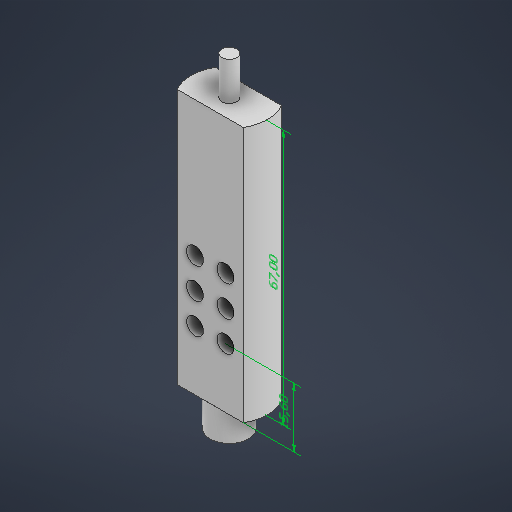
# Autodesk Inventor part: Launcher_shaft
Saved by Autodesk Inventor 2026.1 (Build 301233020, 233B)
## iProperties
Created: 2025-10-31
Part Number: Launcher_shaft
Material: Generic
Document SubType Name: Modeling
Designer: Asus
Density: 1 g/cm^3
Appearance: Default
Author: Asus
Autodesk Inventor part; units mm, degrees
ref_plane "YZ Plane" through (0, 0, 0) normal (1, 0, 0) x (0, 1, 0)
ref_plane "XZ Plane" through (0, 0, 0) normal (0, 1, 0) x (-1, 0, 0)
ref_plane "XY Plane" through (0, 0, 0) normal (0, 0, 1) x (1, 0, 0)
sketch "Sketch1" plane through (0, 0, 0) normal (0, 1, 0) x (-1, 0, 0)
  line L0 (-2.0347, 1.85) -> (2.0347, 1.85)
  line L1 (2.0347, -1.85) -> (-2.0347, -1.85)
  line L2 (-2.0347, 1.85) -> (2.0347, -1.85) construction
  line L3 (2.0347, 1.85) -> (-2.0347, -1.85) construction
  circle A0 centre (0, 0) radius 5
  arc A1 (2.0347, -1.85) -> (2.0347, 1.85) centre (0, 0) ccw
  arc A2 (-2.0347, 1.85) -> (-2.0347, -1.85) centre (0, 0) ccw
  dimension "d2" = 10
  constraints: 8 end point, 4 point on circle, 3 centre point, 2 coincident, 2 midpoint, 1 horizontal, 1 parallel
  measures "d2" diameter of A0
extrude "Extrusion1" add sketch "Sketch1" along normal blind 8
sketch "Sketch2" plane through (0, 8, 0) normal (0, 1, 0) x (1, 0, 0)
  circle A0 centre (0, 0) radius 10
  dimension "d10" = 20
  constraints: 1 centre point, 1 coincident
  measures "d10" diameter of A0
extrude "Extrusion2" add sketch "Sketch2" along normal blind 67
sketch "Sketch3" plane through (0, 75, 0) normal (0, 1, 0) x (1, 0, 0)
  circle A0 centre (0, 0) radius 1.95
  dimension "d7" = 3.9
  constraints: 1 centre point, 1 coincident
  measures "d7" diameter of A0
extrude "Extrusion3" add sketch "Sketch3" along normal blind 10
sketch "Sketch4" plane through (0, 8, 0) normal (0, -1, 0) x (1, 0, 0)
  circle A0 centre (0, 0) radius 5 projected
  line L0 (0, 5) -> (8.6603, 5)
  line L1 (0, 5) -> (-8.6603, 5)
  line L2 (-8.6603, -5) -> (8.6603, -5)
  arc A1 (-8.6603, -5) -> (8.6603, -5) centre (0, 0) ccw
  arc A2 (8.6603, 5) -> (-8.6603, 5) centre (0, 0) ccw
  constraints: 6 end point, 4 point on circle, 2 centre point, 2 horizontal, 1 coincident, 1 parallel, 1 point on line, 1 vertical alignment, 1 other
extrude "Extrusion4" cut sketch "Sketch4" against normal blind 67 contours L2 A1 | L1 A2 L0
sketch "Sketch5" plane through (-8.6603, 8, 5) normal (0, 0, 1) x (1, 0, 0)
  circle A0 centre (4.66, -0.4) radius 2.2
  line L0 (4.66, -0.4) -> (12.66, -0.4) construction
  line L1 (4.66, -0.4) -> (4.66, 67) construction
  line L2 (17.3205, 67) -> (0, 67) projected
  line L3 (4.66, 7.6) -> (4.66, 75) construction
  circle A1 centre (4.66, 7.6) radius 2.2
  line L4 (4.66, 15.6) -> (4.66, 83) construction
  circle A2 centre (4.66, 15.6) radius 2.2
  line L5 (4.66, 23.6) -> (4.66, 91) construction
  circle A3 centre (4.66, 23.6) radius 2.2
  line L6 (4.66, 31.6) -> (4.66, 99) construction
  circle A4 centre (4.66, 31.6) radius 2.2
  line L7 (12.66, -0.4) -> (12.66, 67) construction
  circle A5 centre (12.66, -0.4) radius 2.2
  line L8 (12.66, 7.6) -> (12.66, 75) construction
  circle A6 centre (12.66, 7.6) radius 2.2
  line L9 (12.66, 15.6) -> (12.66, 83) construction
  circle A7 centre (12.66, 15.6) radius 2.2
  line L10 (12.66, 23.6) -> (12.66, 91) construction
  circle A8 centre (12.66, 23.6) radius 2.2
  line L11 (12.66, 31.6) -> (12.66, 99) construction
  circle A9 centre (12.66, 31.6) radius 2.2
  line L12 (8.6603, 0) -> (0, 0) projected
  line L13 (13.6603, -8) -> (3.6603, -8) projected
  point P0 (8.6603, -8)
  dimension "d24" = 8
  dimension "d27" = 8
  dimension "d33" = 7.6
  constraints: 22 end point, 10 centre point, 2 horizontal, 2 vertical, 1 collinear, 1 point on line, 35 other
  measures "d24" distance of L0.start L3.start
  measures "d27" distance of L0.start L7.start
  measures "d33" distance from line of L13 L0.start
extrude "Extrusion5" cut sketch "Sketch5" against normal blind 20.5 contours A2 | A3 | A4 | A7 | A8 | A9
body "Solid1"
